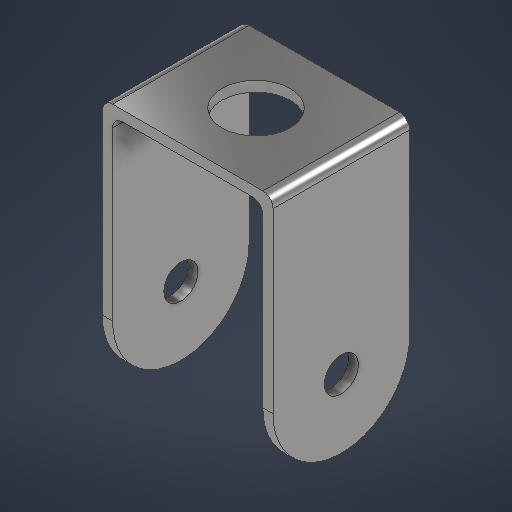
# Autodesk Inventor part: Part1
Saved by Autodesk Inventor 2026 (Build 300175050, 175E)
## iProperties
Created: 2026-05-07
Part Number: Part1
Material: Steel, Carbon
Document SubType Name: Modeling
Designer: Administrator
Density: 7.85 g/cm^3
Appearance: Semi-Polished
Mass: 163.564 g
Surface Area: 153.628 cm^2
Volume: 20.8362 cm^3
Author: Administrator
Autodesk Inventor part; units mm, degrees
ref_plane "YZ Plane" through (0, 0, 0) normal (1, 0, 0) x (0, 1, 0)
ref_plane "XZ Plane" through (0, 0, 0) normal (0, 1, 0) x (-1, 0, 0)
ref_plane "XY Plane" through (0, 0, 0) normal (0, 0, 1) x (1, 0, 0)
sketch "Sketch1" plane through (0, 0, 0) normal (0, 0, 1) x (1, 0, 0)
  line L0 (0, 0) -> (0, 75)
  line L1 (0, 75) -> (50, 75)
  line L2 (50, 75) -> (50, 0)
  line L3 (47, 0) -> (47, 72)
  line L4 (47, 72) -> (3, 72)
  line L5 (3, 72) -> (3, 0)
  line L6 (0, 0) -> (3, 0)
  line L7 (47, 0) -> (50, 0)
  dimension "d0" = 75
  dimension "d1" = 50
  dimension "d2" = 3
  constraints: 16 end point, 4 perpendicular, 1 collinear, 1 horizontal, 1 vertical, 2 other
  measures "d0" distance of L0.start L0.end
  measures "d1" distance of L0.end L1.end
  measures "d2" distance between parallel lines of L1 L4
extrude "Extrusion1" add sketch "Sketch1" along normal mid plane 40
fillet "Fillet1" radius 3 4 edges at (50, 75, 0) (0, 75, 0) (3, 72, 0) (47, 72, 0)
fillet "Fillet2" radius 20 4 edges at (1.5, 0, 20) (48.5, 0, 20) (1.5, 0, -20) (48.5, 0, -20)
sketch "Sketch2" plane through (50, 72, 20) normal (1, 0, 0) x (0, 0, -1)
  arc A0 (0, -52) -> (40, -52) centre (20, -52) ccw projected
  circle A1 centre (20, -52) radius 5
  point P0 (20, -72)
  dimension "d7" = 10
  constraints: 1 centre point, 1 coincident
  measures "d7" diameter of A1
extrude "Extrusion2" cut sketch "Sketch2" against normal through all
sketch "Sketch3" plane through (3, 75, 20) normal (0, 1, 0) x (1, 0, 0)
  circle A0 centre (22, 20) radius 10
  point P0 (-3, 20)
  dimension "d10" = 20
  constraints: 1 centre point
  measures "d10" diameter of A0
extrude "Extrusion3" cut sketch "Sketch3" against normal through all
body "Solid1"
